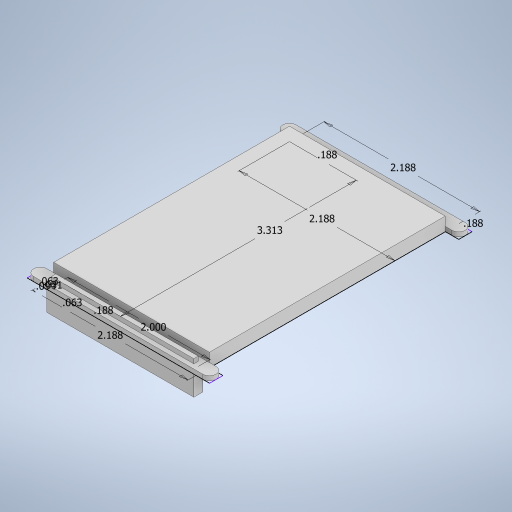
# Autodesk Inventor part: LCD_Display
Saved by Autodesk Inventor 2023 (Build 270158000, 158)
## iProperties
Created: 2022-12-07
Part Number: LCD_Display
Material: Generic
Document SubType Name: Modeling
Designer: spfow
Density: 1 g/cm^3
Appearance: Default
Author: spfow
Autodesk Inventor part; units mm, degrees
ref_plane "YZ Plane" through (0, 0, 0) normal (1, 0, 0) x (0, 1, 0)
ref_plane "XZ Plane" through (0, 0, 0) normal (0, 1, 0) x (-1, 0, 0)
ref_plane "XY Plane" through (0, 0, 0) normal (0, 0, 1) x (1, 0, 0)
sketch "Sketch1" plane through (0, 0, 0) normal (0, 1, 0) x (-1, 0, 0)
  line L0 (0, 0) -> (55.5625, 0)
  line L1 (55.5625, 0) -> (55.5625, -84.1375)
  line L2 (55.5625, -84.1375) -> (0, -84.1375)
  line L3 (0, -84.1375) -> (0, 0)
  line L4 (55.5625, 0) -> (0, 0)
  line L5 (0, 0) -> (0, 4.7625)
  line L6 (0, 4.7625) -> (55.5625, 4.7625)
  line L7 (55.5625, 4.7625) -> (55.5625, 0)
  line L8 (55.5625, -84.1375) -> (0, -84.1375)
  line L9 (0, -84.1375) -> (0, -88.9)
  line L10 (0, -88.9) -> (55.5625, -88.9)
  line L11 (55.5625, -88.9) -> (55.5625, -84.1375)
  line L12 (55.5625, 4.7625) -> (60.325, 4.7625)
  line L13 (55.5625, 1.7145) -> (55.5625, 4.7625)
  line L14 (55.5625, -84.1375) -> (60.325, -84.1375)
  line L15 (60.325, -84.1375) -> (60.325, -88.9)
  line L16 (60.325, -88.9) -> (55.5625, -88.9)
  line L17 (55.5625, -88.9) -> (55.5625, -84.1375)
  line L18 (0, -84.1375) -> (-4.7625, -84.1375)
  line L19 (-4.7625, -84.1375) -> (-4.7625, -88.9)
  line L20 (-4.7625, -88.9) -> (0, -88.9)
  line L21 (0, -88.9) -> (0, -84.1375)
  line L22 (0, 4.7625) -> (-4.7625, 4.7625)
  line L23 (-4.7625, 4.7625) -> (-4.7625, 1.7145)
  line L24 (0, 1.7145) -> (0, 4.7625)
  line L25 (53.1812, 3.175) -> (2.3812, 3.175)
  line L26 (2.3812, 3.175) -> (2.3812, 1.5875)
  line L27 (2.3812, 1.5875) -> (53.1812, 1.5875)
  line L28 (53.1812, 1.5875) -> (53.1812, 3.175)
  line L29 (53.975, 3.9687) -> (1.5875, 3.9687)
  line L30 (1.5875, 3.9687) -> (1.5875, 0.7938)
  line L31 (1.5875, 0.7938) -> (53.975, 0.7938)
  line L32 (53.975, 0.7938) -> (53.975, 3.9687)
  line L33 (60.325, 4.7625) -> (55.5625, 4.7625)
  line L34 (55.5625, 4.7625) -> (55.5625, 0)
  line L35 (55.5625, 0) -> (60.325, 0)
  line L36 (60.325, 0) -> (60.325, 4.7625)
  line L37 (0, 4.7625) -> (-4.7625, 4.7625)
  line L38 (-4.7625, 4.7625) -> (-4.7625, 0)
  line L39 (-4.7625, 0) -> (0, 0)
  line L40 (0, 0) -> (0, 4.7625)
  point P0 (55.5625, 2.3813)
  point P1 (0, -88.9)
  point P2 (-4.7625, 1.7145)
  dimension "d0" = 55.5625
  dimension "d1" = 84.1375
  dimension "d2" = 55.5625
  dimension "d4" = 55.5625
  dimension "d7" = 4.7625
  dimension "d8" = 4.7625
  dimension "d9" = 4.7625
  dimension "d10" = 50.8
  dimension "d12" = 1.5875
  dimension "d13" = 1.5875
  dimension "d14" = 2.3813
  dimension "d15" = 0.7937
  constraints: 82 end point, 19 parallel, 10 horizontal, 10 perpendicular, 3 point on line, 1 midpoint, 3 other
  measures "d0" distance of L1.end L2.end
  measures "d1" distance of L0.end L1.end
  measures "d2" distance of L5.end L6.end
  measures "d4" distance of L10.end L9.end
  measures "d7" distance of L20.end L19.end
  measures "d8" distance between parallel lines of L0 L6
  measures "d9" distance between parallel lines of L10 L2
  measures "d10" distance of L26.end L27.end
  measures "d12" distance of L27.end L25.start
  measures "d13" distance between parallel lines of L6 L25
  measures "d14" distance from line of point (55.563, 2.381) L28
  measures "d15" distance between parallel lines of L28 L32
extrude "Extrusion1" add sketch "Sketch1" along normal blind 4.7625 contours L0 L1 L2 L3
extrude "Extrusion2" add sketch "Sketch1" along normal blind 1.5875 contours L5 L6 L7 L0 | L2 L11 L10 L9 | L9 L20 L19 L18 | L14 L15 L16 L11 | L28 L27 L26 L25 | L32 L31 L30 L29
extrude "Extrusion3" add sketch "Sketch1" along normal blind 1.5875 contours L39 L38 L23 L22 L5 | L7 L12 L36 L35
extrude "Extrusion4" add sketch "Sketch1" along normal blind 3.175 contours L28 L27 L26 L25
extrude "Extrusion5" add sketch "Sketch1" against normal blind 7.9375 contours L28 L27 L26 L25 | L32 L31 L30 L29
fillet "Fillet1" radius 2.3813 8 edges at (-60.325, 0.7937, 4.7625) (-60.325, 0.7937, 0) (4.7625, 0.7937, 4.7625) (4.7625, 0.7937, 0) (4.7625, 0.7937, -84.1375) (4.7625, 0.7937, -88.9) (-60.325, 0.7937, -88.9) (-60.325, 0.7937, -84.1375)
body "Solid1"
